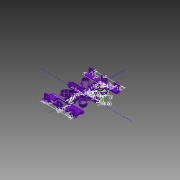
# Autodesk Inventor part: Flex16Test
Saved by Autodesk Inventor 2014 SP1 (Build 180222100, 222)
## iProperties
Created: 2015-02-27
Part Number: Flex16Test
Material: Generic
Document SubType Name: Modeling
Designer: Erin
Density: 1 g/cm^3
Appearance: Default
Author: Erin
Autodesk Inventor part; units mm, degrees
ref_plane "YZ Plane" through (0, 0, 0) normal (1, 0, 0) x (0, 1, 0)
sketch "Block1" plane through (0, 0, 0) normal (0, 0, 1) x (1, 0, 0)
  circle A0 centre (47.029, 24.2723) radius 1.1
  circle A1 centre (75.029, 24.2723) radius 1.1
  line L0 (49.279, 30.4723) -> (72.779, 30.4723)
  line L1 (72.779, 30.4723) -> (72.779, 18.0723)
  line L2 (72.779, 18.0723) -> (49.279, 18.0723)
  line L3 (49.279, 18.0723) -> (49.279, 30.4723)
  line L4 (49.279, 30.4723) -> (44.779, 30.4723)
  line L5 (44.779, 30.4723) -> (44.779, 18.0723)
  line L6 (44.779, 18.0723) -> (49.279, 18.0723)
  line L7 (49.279, 18.0723) -> (49.279, 30.4723)
  line L8 (72.779, 30.4723) -> (77.279, 30.4723)
  line L9 (77.279, 30.4723) -> (77.279, 18.0723)
  line L10 (77.279, 18.0723) -> (72.779, 18.0723)
  line L11 (72.779, 18.0723) -> (72.779, 30.4723)
  line L12 (44.779, 24.2723) -> (77.279, 24.2723) construction
  line L13 (61.029, 30.4723) -> (61.029, 18.0723) construction
  line L14 (47.029, 30.4723) -> (47.029, 18.0723) construction
  line L15 (75.029, 30.4723) -> (75.029, 18.0723) construction
  line L16 (66.779, 30.4723) -> (66.779, 18.0723) construction
  point P0 (60.979, 24.0984)
  dimension "d105" = 23.5
  dimension "d106" = 12.4
  dimension "d107" = 4.5
  dimension "d108" = 4.5
  dimension "d109" = 2.2
  dimension "d110" = 2.2
  dimension "d111" = 2.25
  dimension "d112" = 6
  measures "d105" distance of L1.end L2.end
  measures "d106" distance of L0.end L1.end
  measures "d107" distance of L6.end L5.end
  measures "d108" distance of L9.end L10.end
  measures "d109" diameter of A0
  measures "d110" diameter of A1
  measures "d111" distance between parallel lines of L9 L15
  measures "d112" distance between parallel lines of L16 L1
sketch "Sketch1" plane through (0, 0, 0) normal (0, 0, 1) x (1, 0, 0)
  circle A0 centre (0, 0) radius 7.5
  circle A1 centre (0, 0) radius 10.5
  line L0 (0, 82.8355) -> (0, -64.7276) construction
  line L1 (-84.476, 0) -> (94.8366, 0) construction
  line L2 (6.6657, 3.617) -> (21.9866, 16.4727)
  circle A2 centre (0, 0) radius 13.5
  circle A3 centre (0, 0) radius 16.5
  line L3 (-30, 38.5) -> (30, 38.5)
  line L4 (30, 38.5) -> (30, 31.5)
  line L5 (30, 31.5) -> (-30, 31.5)
  line L6 (-30, 31.5) -> (-30, 38.5)
  line L7 (-30, -47.9) -> (30, -47.9)
  line L8 (30, -47.9) -> (30, -31.5)
  line L9 (30, -31.5) -> (-30, -31.5)
  line L10 (-30, -31.5) -> (-30, -47.9)
  line L11 (21.9866, 16.4727) -> (21.3438, 17.2388)
  line L12 (14.8706, 24.2954) -> (4.892, 12.4033)
  line L13 (4.892, 12.4033) -> (4.126, 13.0461)
  line L14 (4.126, 13.0461) -> (14.1046, 24.9382)
  line L15 (14.1046, 24.9382) -> (14.8706, 24.2954)
  line L16 (3, 13.1273) -> (3.9848, 12.9536)
  line L17 (3.9848, 12.9536) -> (7.2397, 31.4132)
  line L18 (7.2397, 31.4132) -> (6.2549, 31.5868)
  line L19 (6.2549, 31.5868) -> (3, 13.1273)
  circle A4 centre (6.7473, 31.5) radius 1
  line L20 (6.0229, 4.383) -> (6.6657, 3.617)
  line L21 (21.3438, 17.2388) -> (6.0229, 4.383)
  line L22 (6.3443, 4.5) -> (26.3443, 4.5)
  line L23 (26.3443, 4.5) -> (26.3443, 3.5)
  line L24 (26.3443, 3.5) -> (6.3443, 3.5)
  line L25 (6.3443, 3.5) -> (6.3443, 4.5)
  circle A5 centre (6.3443, 4) radius 1
  line L26 (-17.5, 3.5) -> (17.5, 3.5)
  line L27 (17.5, 3.5) -> (17.5, -3.5)
  line L28 (17.5, -3.5) -> (-17.5, -3.5)
  line L29 (-17.5, -3.5) -> (-17.5, 3.5)
  line L30 (12.2251, 21.1426) -> (5.147, 12.7072)
  line L31 (15.5173, 20.8067) -> (17.8844, 16.4197)
  line L32 (17.4099, 13.9378) -> (10.9977, 8.5573)
  line L33 (8.9078, 8.2583) -> (5.8748, 9.5905)
  arc A6 (15.5173, 20.8067) -> (12.2251, 21.1426) centre (13.7572, 19.857) ccw
  arc A7 (17.4099, 13.9378) -> (17.8844, 16.4197) centre (16.1243, 15.4699) ccw
  line L34 (13.0831, 9.0018) -> (19.7338, 14.5824)
  line L35 (22.7883, 13.9836) -> (26.2443, 7.4333)
  line L36 (24.4754, 4.5) -> (14.8803, 4.5)
  line L37 (13.1114, 5.5667) -> (12.5997, 6.5364)
  arc A8 (22.7883, 13.9836) -> (19.7338, 14.5824) centre (21.0194, 13.0503) ccw
  arc A9 (24.4754, 4.5) -> (26.2443, 7.4333) centre (24.4754, 6.5) ccw
  arc A10 (13.1114, 5.5667) -> (14.8803, 4.5) centre (14.8803, 6.5) ccw
  arc A11 (13.0831, 9.0018) -> (12.5997, 6.5364) centre (14.3686, 7.4697) ccw
  arc A12 (5.147, 12.7072) -> (5.8748, 9.5905) centre (6.6791, 11.4217) ccw
  arc A13 (8.9078, 8.2583) -> (10.9977, 8.5573) centre (9.7121, 10.0894) ccw
  line L38 (7.718, 4.5) -> (14.2853, 10.0106)
  line L39 (15.0489, 9.8609) -> (17.4905, 5.2333)
  line L40 (17.0482, 4.5) -> (7.718, 4.5)
  arc A14 (15.0489, 9.8609) -> (14.2853, 10.0106) centre (14.6067, 9.6276) ccw
  arc A15 (17.0482, 4.5) -> (17.4905, 5.2333) centre (17.0482, 5) ccw
  arc A16 (21.3438, 17.2388) -> (14.8706, 24.2954) centre (18.1072, 20.7671) ccw
  arc A17 (21.9866, 16.4727) -> (14.1046, 24.9382) centre (18.0456, 20.7055) ccw
  arc A18 (29.7318, 0) -> (26.3443, 3.5) centre (23.6026, -2.5429) ccw
  arc A19 (30.8471, 0) -> (26.3443, 4.5) centre (23.9388, -2.4098) ccw
  line L41 (29.7318, 0) -> (30.8471, 0)
  line L42 (0, 0.5) -> (30.8471, 0.5)
  line L43 (30.8471, 0.5) -> (30.8471, -0.5)
  line L44 (30.8471, -0.5) -> (0, -0.5)
  line L45 (0, -0.5) -> (0, 0.5)
  circle A20 centre (30.2894, 0) radius 1
  circle A21 centre (0, 35) radius 1.25
  circle A22 centre (7, 35) radius 1.25
  circle A23 centre (14, 35) radius 1.25
  circle A24 centre (-7, 35) radius 1.25
  circle A25 centre (0, 35) radius 1.25
  circle A26 centre (7, 35) radius 1.25
  circle A27 centre (-14, 35) radius 1.25
  circle A28 centre (-7, 35) radius 1.25
  circle A29 centre (0, 35) radius 1.25
  line L46 (-30, -47.9) -> (-20, -47.9)
  line L47 (-20, -47.9) -> (-20, -49.9)
  line L48 (-20, -49.9) -> (-30, -49.9)
  line L49 (-30, -49.9) -> (-30, -47.9)
  line L50 (-5, -47.9) -> (5, -47.9)
  line L51 (5, -47.9) -> (5, -49.9)
  line L52 (5, -49.9) -> (-5, -49.9)
  line L53 (-5, -49.9) -> (-5, -47.9)
  line L54 (30, -47.9) -> (20, -47.9)
  line L55 (20, -47.9) -> (20, -49.9)
  line L56 (20, -49.9) -> (30, -49.9)
  line L57 (30, -49.9) -> (30, -47.9)
  line L58 (-30, 38.5) -> (-20, 38.5)
  line L59 (-20, 38.5) -> (-20, 40.5)
  line L60 (-20, 40.5) -> (-30, 40.5)
  line L61 (-30, 40.5) -> (-30, 38.5)
  line L62 (-5, 40.5) -> (5, 40.5)
  line L63 (5, 40.5) -> (5, 38.5)
  line L64 (5, 38.5) -> (-5, 38.5)
  line L65 (-5, 38.5) -> (-5, 40.5)
  line L66 (30, 38.5) -> (20, 38.5)
  line L67 (20, 38.5) -> (20, 40.5)
  line L68 (20, 40.5) -> (30, 40.5)
  line L69 (30, 40.5) -> (30, 38.5)
  circle A30 centre (-19.75, -39.7) radius 1.1
  circle A31 centre (8.25, -39.7) radius 1.1
  line L70 (-17.5, -33.5) -> (6, -33.5)
  line L71 (6, -33.5) -> (6, -45.9)
  line L72 (6, -45.9) -> (-17.5, -45.9)
  line L73 (-17.5, -45.9) -> (-17.5, -33.5)
  line L74 (-17.5, -33.5) -> (-22, -33.5)
  line L75 (-22, -33.5) -> (-22, -45.9)
  line L76 (-22, -45.9) -> (-17.5, -45.9)
  line L77 (-17.5, -45.9) -> (-17.5, -33.5)
  line L78 (6, -33.5) -> (10.5, -33.5)
  line L79 (10.5, -33.5) -> (10.5, -45.9)
  line L80 (10.5, -45.9) -> (6, -45.9)
  line L81 (6, -45.9) -> (6, -33.5)
  line L82 (-22, -39.7) -> (10.5, -39.7) construction
  line L83 (-5.75, -33.5) -> (-5.75, -45.9) construction
  line L84 (-19.75, -33.5) -> (-19.75, -45.9) construction
  line L85 (8.25, -33.5) -> (8.25, -45.9) construction
  line L86 (0, -33.5) -> (0, -45.9) construction
  point P0 (4.509, 12.7247)
  point P1 (3.4924, 13.0404)
  point P2 (0, 38.5)
  point P3 (0, -31.5)
  point P4 (17.5, 0)
  point P5 (3.4321, 10.6635)
  point P6 (18.6583, 14.9854)
  point P7 (11.8464, 7.9642)
  point P8 (21.632, 16.1752)
  point P9 (27.792, 4.5)
  point P10 (13.6742, 4.5)
  point P11 (14.7598, 10.4088)
  point P12 (17.8774, 4.5)
  point P13 (0, -49.9)
  point P14 (0, 40.5)
  point P15 (30, 35)
  dimension "d0" = 15
  dimension "d1" = 3
  dimension "d4" = 40
  dimension "d5" = 3
  dimension "d6" = 3
  dimension "d8" = 1
  dimension "d15" = 1
  dimension "d18" = 1
  dimension "d20" = 3
  dimension "d21" = 10
  dimension "d23" = 2
  dimension "d27" = 4
  dimension "d28" = 20
  dimension "d31" = 60
  dimension "d32" = 60
  dimension "d33" = 15
  dimension "d34" = 7
  dimension "d36" = 20
  dimension "d37" = 1
  dimension "d38" = 2
  dimension "d43" = 15
  dimension "d51" = 2
  dimension "d58" = 2
  dimension "d59" = 2
  dimension "d60" = 2
  dimension "d63" = 1
  dimension "d64" = 1
  dimension "d65" = 0.5
  dimension "d76" = 1
  dimension "d77" = 2
  dimension "d94" = 2.5
  dimension "d97" = 7
  dimension "d100" = 7
  dimension "d113" = 2
  dimension "d114" = 2
  dimension "d115" = 10
  dimension "d116" = 2
  dimension "d117" = 10
  dimension "d118" = 2
  dimension "d119" = 10
  dimension "d120" = 2
  dimension "d121" = 10
  dimension "d122" = 2
  dimension "d123" = 10
  dimension "d124" = 2
  dimension "d125" = 10
  dimension "d141" = 2
  dimension "d142" = 50
  constraints: 140 end point, 31 point on line, 30 point on circle, 29 centre point, 28 parallel, 20 tangent, 18 perpendicular, 14 horizontal, 14 midpoint, 5 coincident, 5 collinear, 5 equal radius, 4 vertical alignment, 3 vertical, 2 horizontal alignment, 19 other
  measures "d4" angle of L1 L2
  measures "d5" radial gap between concentric circles of A1 A2
  measures "d6" radial gap between concentric circles of A2 A3
  measures "d8" distance of L2.end L11.end
  measures "d15" distance of L12.end L13.end
  measures "d18" distance of L18.end L17.end
  measures "d20" distance from line of L16.start L0
  measures "d21" angle of L19 L0
  measures "d23" diameter of A4
  measures "d27" distance from line of point (6.344, 4) L1
  measures "d28" distance of L2.start L2.end
  measures "d31" distance of L3.start L3.end
  measures "d32" distance of L7.start L7.end
  measures "d33" distance edge to line of A3 L9
  measures "d34" distance of L5.end L3.start
  measures "d36" distance of L23.end L24.end
  measures "d37" distance of L22.end L23.end
  measures "d38" diameter of A5
  measures "d43" distance edge to line of A3 L5
  measures "d51" radius of A6
  measures "d58" radius of A8
  measures "d59" radius of A11
  measures "d60" radius of A12
  measures "d63" distance edge to line of A3 L29
  measures "d64" distance edge to line of A3 L27
  measures "d65" radius of A14
  measures "d76" distance of L42.end L43.end
  measures "d77" diameter of A20
  measures "d94" diameter of A21
  measures "d97" distance of A21.centre A22.centre
  measures "d100" distance of A21.centre A24.centre
  measures "d115" distance of L47.end L48.end
  measures "d116" distance of L46.end L47.end
  measures "d117" distance of L51.end L52.end
  measures "d118" distance of L50.end L51.end
  measures "d119" distance of L56.end L55.end
  measures "d120" distance of L55.end L54.end
  measures "d121" distance of L60.end L59.end
  measures "d122" distance of L59.end L58.end
  measures "d123" distance of L63.end L64.end
  measures "d124" distance of L62.end L63.end
  measures "d125" distance of L67.end L68.end
  measures "d141" distance of L66.end L67.end
  measures "d142" angle of L1 L12
extrude "Extrusion2" add sketch "Sketch1" along normal blind 5 contours A0 L42 A1 L44 | A0 A5 L24 A1 L42 | L44 A1 L28 A0 | L28 A1 A0 | A5 L2 L22 A1 L24 | L42 A3 L44 A2 | A2 L24 A3 L42 | L28 A1 L26 A0 | L44 A3 L28 A2 | L25 L22 A5 L2 L20 | A0 L26 A1 L21 A5 | L22 L2 A1 | A2 L22 A3 L24 | L28 A3 A2 | L21 A1 L2 L22 A5 | A5 L22 L2 | A2 L2 A11 L37 A10 L22 | L28 A3 L26 A2 | L26 A3 L19 A2 | A2 L21 A3 L2 | A10 L37 A11 L2 A3 L22 | A2 A13 L21 | L19 A3 L17 L16 A2 | A2 A12 L12 A3 L21 A13 | L16 L17 A3 L14 L13 A2 | A2 L12 A12 | L13 L14 A3 L12 A2
extrude "Extrusion3" cut sketch "Sketch1" along normal blind 10 contours A0 L44 L45 L42 | A0 L42 A1 L44 | L42 L45 L44 A0 L28 L26 A5 | A0 A5 L24 A1 L42 | L44 A1 L28 A0 | A5 L26 L24 A0 | A0 L24 A5 | L42 A2 L44 A1 | A1 L24 A2 L42 | L44 A2 L28 A1 | L42 A3 L44 A2 | A2 L24 A3 L42 | L28 A1 L26 A0 | L44 A3 L28 A2 | L42 L27 L44 A3 | A3 L24 L27 L42 | L28 A2 L26 A1 | L44 L27 L28 A3 | L28 A3 L26 A2 | L28 L29 L26 A3
extrude "Extrusion4" cut sketch "Sketch1" along normal blind 10 contours L22 L2 A1 | A1 L2 A2 L22 | A2 L2 A11 L37 A10 L22 | A10 L37 A11 L2 A3 L22 | A3 L2 A14 L39 A15 L22 | A13 L33 A12 A2 | A2 A12 L12 A3 L21 A13 | A3 L12 A6 L31 A7 L21
extrude "Extrusion1" add sketch "Sketch1" along normal blind 5 contours A5 L26 L24 A0 | A0 L24 A5 | L24 L25 A0 | A0 L20 L2 A5 L24 | A5 A0 L21 L20 L25 L26 | A5 L2 L22 A1 L24 | A1 L22 A2 L24 | L20 L21 A0 | L25 L22 A5 L2 L20 | A0 L21 A5 L22 L25 | A5 L21 A0 | A2 L22 A3 L24 | L21 A1 L2 L22 A5 | A5 L22 L2 | A1 L21 A2 L2 | A3 L22 L23 L24 | A2 L21 A3 L2 | L19 A3 L17 L16 A2 | A2 L16 L19 | A3 L21 L11 L2 | L23 A19 A20 A18 | L42 A19 L41 A18 | A18 A20 A19 L42 | L19 A4 L17 A3 | L13 L14 A3 L12 A2 | A2 L12 L13 | A4 L5 L19 | L19 L5 L18 L17 A4 | A3 L14 L15 L12 | L17 L18 L5 A4 | L19 L18 L5 | L5 A4 L18 L19 | L11 A16 L15 A17
mirror "Mirror1" about plane through (0, 0, 0) normal (1, 0, 0) of "Extrusion4", "Extrusion1"
mirror "Mirror2" about plane through (0, 0, 0) normal (0, 1, 0) of "Extrusion1", "Mirror1", "Extrusion4"
extrude "Extrusion5" add sketch "Sketch1" along normal blind 5 contours A0 L44 L45 L42 | A0 L42 A1 L44 | L42 A2 L44 A1 | L42 A3 L44 A2 | L42 L27 L44 A3 | L42 A20 L44 L27 | A20 A18 L42 | L42 A18 L41 L43 L44 A20 | L44 L43 L42 A19 A20 | L42 A19 L41 A18 | A18 A20 A19 L42 | L42 L43 A19
sketch "Sketch2" plane through (0, 0, 0) normal (0, 0, 1) x (1, 0, 0)
  circle A0 centre (-21.4191, 24.5638) radius 2.5
  circle A1 centre (-28.9868, 35.6578) radius 5
  circle A2 centre (-30.5786, 0) radius 2.5
  circle A3 centre (-11.2882, 38.9668) radius 2.5
  circle A4 centre (-9.7821, 19.1136) radius 2.5
  circle A5 centre (-19.647, 15.1079) radius 2.5
  circle A6 centre (-5.9433, 25.7064) radius 2.5
  point P0 (0, 0)
  dimension "d66" = 5
  dimension "d67" = 10
  dimension "d69" = 5
  dimension "d71" = 5
  dimension "d72" = 5
  dimension "d73" = 5
  dimension "d148" = 5
  constraints: 7 centre point
  measures "d66" diameter of A0
  measures "d67" diameter of A1
  measures "d69" diameter of A2
  measures "d71" diameter of A3
  measures "d72" diameter of A4
  measures "d73" diameter of A5
  measures "d148" diameter of A6
extrude "Extrusion6" add sketch "Sketch2" along normal blind 0.3
mirror "Mirror3" about plane through (0, 0, 0) normal (1, 0, 0) of "Extrusion6"
mirror "Mirror4" about plane through (0, 0, 0) normal (0, 1, 0) of "Extrusion6", "Mirror3"
mirror "Mirror5" about plane through (0, 0, 0) normal (1, 0, 0) of "Extrusion5"
sketch "Sketch3" plane through (0, 0, 0) normal (1, 0, 0) x (0, 1, 0)
  line L0 (-70.3552, 2.5) -> (72.4069, 2.5) construction
  circle A0 centre (-28.0293, 2.5) radius 1.25
  circle A1 centre (-22.3345, 2.5) radius 1.25
  point P0 (0, 0)
  dimension "d78" = 2.5
  dimension "d79" = 2.5
  dimension "d82" = 2.5
  constraints: 2 centre point, 2 end point, 2 point on line, 1 horizontal
  measures "d78" distance from line of point (0, 0) L0
  measures "d79" diameter of A0
  measures "d82" diameter of A1
extrude "Extrusion7" cut sketch "Sketch3" along normal mid plane 20
pattern_circular "Circular Pattern1" count 8 over 360 about axis through (0, 0, -10) along (0, 0, 1) of "Extrusion7"
sketch "Sketch4" plane through (0, 0, 0) normal (0, 1, 0) x (-1, 0, 0)
  line L0 (-58.2756, 2.5) -> (59.4862, 2.5) construction
  circle A0 centre (-15, 2.5) radius 1.25
  circle A1 centre (15, 2.5) radius 1.25
  line L1 (0, 12.237) -> (0, -7.8921) construction
  circle A2 centre (0, 2.5) radius 1.25
  circle A3 centre (-7.5, 2.5) radius 1.25
  circle A4 centre (7.5, 2.5) radius 1.25
  point P0 (0, 0)
  dimension "d86" = 2.5
  dimension "d87" = 2.5
  dimension "d88" = 2.5
  dimension "d89" = 15
  dimension "d90" = 15
  dimension "d91" = 2.5
  dimension "d143" = 2.5
  dimension "d144" = 7.5
  dimension "d145" = 2.5
  dimension "d146" = 7.5
  constraints: 6 point on line, 5 centre point, 4 end point, 1 horizontal, 1 perpendicular, 1 vertical
  measures "d86" distance from line of point (0, 0) L0
  measures "d87" diameter of A0
  measures "d88" diameter of A1
  measures "d89" distance from line of L1 A0.centre
  measures "d90" distance from line of A1.centre L1
  measures "d91" diameter of A2
  measures "d143" diameter of A3
  measures "d144" distance from line of L1 A3.centre
  measures "d145" diameter of A4
  measures "d146" distance from line of A4.centre L1
extrude "Extrusion8" cut sketch "Sketch4" along normal mid plane 10
extrude "Extrusion9" add sketch "Sketch1" along normal blind 2 contours L19 L18 L5 | L5 A4 L18 L19 | L5 L6 L3 L4 A4 | L10 L9 L8 L7 | L73 L76 L75 L74 | L78 L79 L80 L71
extrude "Extrusion10" add sketch "Sketch1" along normal blind 12 contours L61 L60 L59 L3 | L3 L67 L68 L69 | L65 L62 L63 L3 | L7 L47 L48 L49 | L7 L51 L52 L53 | L57 L56 L55 L7
ref_plane "Work Plane1" through (-30, 38.5, 2) normal (0, -1, 0) x (1, 0, 0)
sketch "Sketch5" plane through (-30, 38.5, 2) normal (0, -1, 0) x (1, 0, 0)
  circle A0 centre (5, 5) radius 2.25
  circle A1 centre (30, 5) radius 2.25
  line L0 (57.7404, -2) -> (50, -2) projected
  line L1 (50, -2) -> (50, 10) projected
  line L2 (60, 10) -> (50, 10) projected
  line L3 (60, -1.7) -> (60, 10) projected
  line L4 (25, -2) -> (35, -2) projected
  line L5 (25, -2) -> (25, 10) projected
  line L6 (35, 10) -> (25, 10) projected
  line L7 (35, -2) -> (35, 10) projected
  circle A2 centre (55, 5) radius 2.25
  line L8 (57.7404, -2) -> (57.7404, -1.7) projected
  line L9 (57.7404, -1.7) -> (60, -1.7) projected
  point P0 (30, -2)
  point P1 (30, 10)
  point P2 (55, 10)
  dimension "d129" = 4.5
  dimension "d130" = 4.5
  dimension "d131" = 4.5
  constraints: 3 centre point, 2 midpoint, 2 vertical alignment
  measures "d129" diameter of A0
  measures "d130" diameter of A1
  measures "d131" diameter of A2
extrude "Extrusion11" cut sketch "Sketch5" against normal blind 3 contours A0 | A1 | A2
ref_plane "Work Plane2" through (-30, -47.9, 2) normal (0, 1, 0) x (1, 0, 0)
sketch "Sketch6" plane through (-30, -47.9, 2) normal (0, 1, 0) x (1, 0, 0)
  line L0 (25, 2) -> (35, 2) projected
  line L1 (35, 2) -> (35, -10) projected
  line L2 (25, -10) -> (35, -10) projected
  line L3 (25, 2) -> (25, -10) projected
  line L4 (50, 2) -> (60, 2) projected
  line L5 (60, 2) -> (60, -10) projected
  line L6 (50, -10) -> (60, -10) projected
  line L7 (50, 2) -> (50, -10) projected
  circle A0 centre (5, -5) radius 2.25
  circle A1 centre (30, -5) radius 2.25
  circle A2 centre (55, -5) radius 2.25
  line L8 (35, -10) -> (25, -10) projected
  line L9 (60, -10) -> (50, -10) projected
  point P0 (30, 2)
  point P1 (30, -10)
  point P2 (55, -10)
  dimension "d135" = 4.5
  dimension "d136" = 4.5
  dimension "d137" = 4.5
  constraints: 3 centre point, 2 midpoint, 2 vertical alignment
  measures "d135" diameter of A0
  measures "d136" diameter of A1
  measures "d137" diameter of A2
extrude "Extrusion12" cut sketch "Sketch6" against normal blind 3 contours A0 | A1 | A2
fillet "Fillet1" radius 3 12 edges at (30, -48.9, 12) (20, -48.9, 12) (5, -48.9, 12) (-5, -48.9, 12) (-20, -48.9, 12) (-30, -48.9, 12) (30, 39.5, 12) (20, 39.5, 12) (5, 39.5, 12) (-5, 39.5, 12) (-20, 39.5, 12) (-30, 39.5, 12)
sketch "Sketch7" plane through (0, 0, 0) normal (0, 0, 1) x (1, 0, 0)
  circle A0 centre (-28.5008, -48.3965) radius 5
  circle A1 centre (28.3788, -48.3965) radius 5
  point P0 (0, 0)
  dimension "d149" = 10
  dimension "d150" = 10
  constraints: 2 centre point
  measures "d149" diameter of A0
  measures "d150" diameter of A1
extrude "Extrusion13" add sketch "Sketch7" along normal blind 0.3
equation "\"d8\" = flex_w"
equation "\"d15\" = flex_w"
equation "\"d18\" = flex_w"
equation "\"d23\" = flex_b"
equation "\"d37\" = flex_w"
equation "\"d38\" = flex_b"
equation "\"thickness\" = 5"
equation "\"screw\" = 4.5"
equation "\"flex_w\" = 1"
equation "\"flex_b\" = 2"
body "Solid1"
